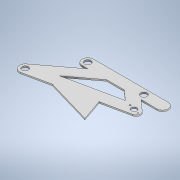
# Autodesk Inventor part: intake-1
Saved by Autodesk Inventor 2022 (Build 260153000, 153)
## iProperties
Created: 2023-01-10
Part Number: intake-1
Material: Generic
Document SubType Name: Modeling
Designer: s135320
Density: 1 g/cm^3
Appearance: Default
Author: s135320
Autodesk Inventor part; units mm, degrees
ref_plane "YZ Plane" through (0, 0, 0) normal (1, 0, 0) x (0, 1, 0)
ref_plane "XZ Plane" through (0, 0, 0) normal (0, 1, 0) x (-1, 0, 0)
ref_plane "XY Plane" through (0, 0, 0) normal (0, 0, 1) x (1, 0, 0)
sketch "Sketch1" plane through (0, 0, 0) normal (0, 1, 0) x (-1, 0, 0)
  line L0 (0, 0) -> (254, 0)
  line L1 (0, -25.4) -> (254, -25.4)
  line L2 (0, 25.4) -> (254, 25.4)
  circle A0 centre (254, 0) radius 25.4
  circle A1 centre (0, 0) radius 25.4
  circle A2 centre (254, 0) radius 14.2875
  circle A3 centre (0, 0) radius 14.2875
  line L3 (76.2, 0) -> (-84.1335, 0)
  line L4 (121.5695, -25.4) -> (-84.1335, -25.4)
  line L5 (40.7781, 25.4) -> (-84.1335, 25.4)
  circle A4 centre (-84.1335, 0) radius 25.4
  line L6 (152.4, 0) -> (371.644, 165.4814)
  line L7 (143.8902, 25.4) -> (356.342, 185.7548)
  line L8 (228.214, 25.4) -> (386.946, 145.208)
  circle A5 centre (371.644, 165.4814) radius 25.4
  circle A6 centre (371.644, 165.4814) radius 14.2875
  circle A7 centre (-34.5114, 79.1283) radius 25.4
  line L9 (53.0811, 0) -> (-34.5114, 79.1283)
  line L10 (13.4025, 70.0738) -> (8.7814, 74.2485)
  line L11 (-4.2871, 17.5951) -> (-21.5461, 33.1863)
  line L12 (-9.1867, 81.0827) -> (-4.2871, 17.5951)
  line L13 (-17.4847, 97.9764) -> (13.4025, 70.0738)
  line L14 (-34.5114, 79.1283) -> (371.644, 165.4814)
  line L15 (366.3617, 190.3261) -> (-88.4526, 93.6275)
  line L16 (-88.4526, 93.6275) -> (19.2621, -3.6785)
  line L17 (409.5559, 199.5096) -> (-88.4526, 93.6275)
  line L18 (-88.4526, 93.6275) -> (-12.9269, 25.4)
  line L19 (419.8284, 149.7582) -> (19.4297, 64.629)
  line L20 (19.4297, 64.629) -> (62.855, 25.4)
  circle A8 centre (-34.5114, 79.1283) radius 12.7
  line L21 (19.4297, 64.629) -> (-88.4526, 93.6275)
  circle A9 centre (-59.0407, 85.7217) radius 3.4925
  circle A10 centre (-9.9821, 72.5349) radius 3.4925
  line L22 (99.5982, 0) -> (99.5982, -97.1111)
  line L23 (99.5982, -97.1111) -> (33.9277, 0)
  line L24 (99.5982, -97.1111) -> (168.3997, 0)
  line L25 (197.5982, 128.4774) -> (41.1424, 225.5805)
  line L26 (41.1424, 225.5805) -> (83.0141, 104.1155)
  line L27 (41.1424, 225.5805) -> (300.5341, 150.3627)
  point P0 (107.1023, -119.4279)
  point P1 (121.5695, -25.4)
  point P2 (2.9551, -25.4)
  point P3 (143.8902, 25.4)
  point P4 (258.2652, 25.0393)
  point P5 (0, 25.4)
  point P6 (16.3526, 37.9742)
  point P7 (0.338, 25.4)
  point P8 (70.7471, 25.4)
  point P9 (4.9006, 69.9742)
  point P10 (-10.4414, 23.1547)
  point P11 (17.5299, 80.8522)
  point P12 (265.0526, 116.8512)
  point P13 (396.2371, 108.5044)
  point P14 (-39.7937, 103.973)
  point P15 (-57.9044, 89.0242)
  point P16 (-51.5382, 60.2802)
  point P17 (-59.7133, 82.2946)
  point P18 (20.6525, 89.1934)
  point P19 (16.5095, 73.5132)
  point P20 (-9.3095, 75.962)
  point P21 (-15.6634, 62.1015)
  point P22 (160.2581, 29.4846)
  point P23 (-11.1184, 69.2324)
  point P24 (382.4437, 141.8098)
  point P25 (376.9262, 140.6367)
  point P26 (323.7481, 129.3305)
  point P27 (186.0521, 25.4)
  point P28 (24.9641, 25.4)
  point P29 (-4.2871, 17.5951)
  point P30 (-12.9269, 25.4)
  point P31 (4.4913, 25.4)
  point P32 (231.3112, 11.4183)
  point P33 (277.9303, 8.5148)
  point P34 (351.3706, 150.1794)
  point P35 (312.9484, 153.0021)
  point P36 (346.7993, 160.1992)
  point P37 (-88.4526, 93.6275)
  point P38 (-2.1293, 19.9838)
  point P39 (-7.1267, 54.3898)
  point P40 (-9.6667, 84.4105)
  point P41 (371.644, 165.4814)
  point P42 (278.63, 6.2067)
  point P43 (230.4586, 9.5373)
  point P44 (-4.8895, 25.4)
  point P45 (60.8476, 25.4)
  point P46 (229.1391, 5.2053)
  point P47 (-12.9269, 25.4)
  point P48 (1.0288, 25.4)
  point P49 (-4.8534, 24.932)
  point P50 (-87.4545, 179.42)
  point P51 (74.6737, 128.31)
  point P52 (248.8661, 165.3452)
  dimension "d0" = 25.4
  dimension "d1" = 25.4
  dimension "d2" = 28.575
  dimension "d3" = 28.575
  dimension "d6" = 254
  dimension "d7" = 76.2
  dimension "d8" = 25.4
  dimension "d9" = 25.4
  dimension "d11" = 50.8
  dimension "d13" = 25.4
  dimension "d14" = 25.4
  dimension "d15" = 50.8
  dimension "d16" = 101.6
  dimension "d18" = 28.575
  dimension "d23" = 50.8
  dimension "d24" = 25.4
  dimension "d25" = 25.4
  dimension "d26" = 25.4
  dimension "d27" = 25.4
  dimension "d28" = 25.4
  dimension "d29" = 25.4
  dimension "d30" = 6.985
  dimension "d31" = 6.985
  constraints: 56 end point, 15 point on line, 13 point on circle, 11 centre point, 8 coincident, 6 parallel, 4 tangent, 2 horizontal, 1 vertical, 3 other
  measures "d0" distance between parallel lines of L0 L2
  measures "d1" distance between parallel lines of L1 L0
  measures "d2" diameter of A3
  measures "d3" diameter of A2
  measures "d6" distance of L0.start L0.end
  measures "d7" distance of L0.start L3.start
  measures "d8" distance between parallel lines of L3 L4
  measures "d9" distance between parallel lines of L3 L5
  measures "d11" diameter of A4
  measures "d13" distance between parallel lines of L6 L7
  measures "d14" distance between parallel lines of L6 L8
  measures "d15" diameter of A5
  measures "d16" distance of L0.end L6.start
  measures "d18" diameter of A6
  measures "d23" diameter of A7
  measures "d24" distance between parallel lines of L9 L10
  measures "d25" distance between parallel lines of L9 L11
  measures "d26" distance between parallel lines of L14 L15
  measures "d27" distance between parallel lines of L14 L17
  measures "d28" distance between parallel lines of L14 L19
  measures "d29" diameter of A8
  measures "d30" diameter of A9
  measures "d31" diameter of A10
extrude "Extrusion1" add sketch "Sketch1" along normal blind 6.35 contours L3 A3 L16 L0 | L0 A3 L3 | A3 L16 L0 | L0 A1 L3 A3 | L3 A1 L11 L16 A3 | L16 A3 L12 A1 L0 | L16 A3 | L3 A4 L5 L11 A1 | A1 L4 A4 L3 | A1 L2 L9 L0 | L0 L23 L1 A1 | L11 A1 L12 | L11 L5 L12 A1 | A4 | L0 L22 L1 L23 | L5 L12 L9 L2 | A1 L12 L5 | L11 L16 A7 L9 L12 L5 | L9 L2 L6 L0 | L9 L12 A10 L21 L20 L2 | L22 L0 L24 L1 | L9 A7 A10 L12 | L16 L21 A9 A7 | A7 A9 L21 A8 L9 | L24 L0 A0 L1 | L20 L19 L7 L2 | L9 A8 L21 A10 A7 | A10 A7 L21 L12 | L12 L21 A10 | A9 L21 A7 | A7 L21 A9 | L15 A7 A9 L21 | L6 L2 A0 L0 | A2 | A0 | L7 L19 L6 L2 | L21 A10 L12 A7 L14 L7 L19 | A10 L21 A7 | A8 L21 L9 | L9 L21 A8 | L21 A7 A10 L12 | L12 A10 L21 | L21 A9 A7 | A7 A9 L21 | A9 A7 L14 A8 L21 | L15 L26 L14 L13 A7 | L6 L19 L8 L2 | L7 L14 A5 L6 L19 | L21 A10 A7 | L21 A8 L14 A7 A10 | L21 A8 L14 | L14 A8 L21 | A10 A7 L12 | L13 L14 A7 | L26 L25 L15 | L15 L25 L14 L26 | L6 A5 L19 | L14 L27 L15 A5 L7 | L7 A5 L14 | L25 L27 L15 | L15 L27 L14 L25 | L19 A5 L8 | A5 L14 A6 L6 | L6 A6 L14 A5 | A6 L14 L6 | L6 L14 A6
extrude "Extrusion2" cut sketch "Sketch1" along normal through all contours L3 A3 L16 L0 | L0 A3 L3 | L16 A3 | L20 L19 L7 L2 | A10 A7 L21 L12 | L12 L21 A10 | A7 L21 A9 | A2 | A10 L21 A7 | A8 L21 L9 | L9 L21 A8 | L21 A7 A10 L12 | L12 A10 L21 | A7 A9 L21 | L21 A10 A7 | L21 A8 L14 | L14 A8 L21 | A6 L14 L6 | L6 L14 A6 picked at (-58.0988, 84.8098) picked at (-57.7672, 86.0943)
fillet "Fillet2" radius 19.05 1 edges at (88.4526, 3.175, 93.6275)
equation "\"d0\" = d1"
body "Solid1"
